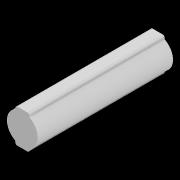
# Autodesk Inventor part: Axel_parametriserad_03
Saved by Autodesk Inventor 2020 (Build 240168000, 168)
## iProperties
Created: 2020-11-22
Part Number: Axel_parametriserad_03
Material: Generic
Document SubType Name: Modeling
Designer: Gottfrid
Density: 1 g/cm^3
Appearance: Default
Author: Gottfrid
Autodesk Inventor part; units mm, degrees
ref_plane "YZ Plane" through (0, 0, 0) normal (1, 0, 0) x (0, 1, 0)
ref_plane "XZ Plane" through (0, 0, 0) normal (0, 1, 0) x (-1, 0, 0)
ref_plane "XY Plane" through (0, 0, 0) normal (0, 0, 1) x (1, 0, 0)
sketch "Sketch1" plane through (0, 0, 0) normal (0, 0, 1) x (1, 0, 0)
  circle A0 centre (0, 0) radius 3.4
  line L0 (1.1333, -3.7357) -> (-1.1333, -3.7357)
  line L1 (-1.5333, -3.3357) -> (-1.5333, 3.3357)
  line L2 (-1.1333, 3.7357) -> (1.1333, 3.7357)
  line L3 (1.5333, 3.3357) -> (1.5333, -3.3357)
  line L4 (1.5333, -3.7357) -> (-1.5333, 3.7357) construction
  line L5 (-1.5333, -3.7357) -> (1.5333, 3.7357) construction
  arc A1 (-1.1333, 3.7357) -> (-1.5333, 3.3357) centre (-1.1333, 3.3357) ccw
  arc A2 (1.5333, 3.3357) -> (1.1333, 3.7357) centre (1.1333, 3.3357) ccw
  arc A3 (1.1333, -3.7357) -> (1.5333, -3.3357) centre (1.1333, -3.3357) ccw
  arc A4 (-1.5333, -3.3357) -> (-1.1333, -3.7357) centre (-1.1333, -3.3357) ccw
  point P0 (-1.5333, 3.0346)
  point P1 (-1.5333, -3.0346)
  point P2 (1.5333, -3.0346)
  point P3 (1.5333, 3.0346)
  point P4 (-0.9416, 2.2076)
  point P5 (-0.9416, -2.2076)
  point P6 (0.9416, -2.2076)
  point P7 (0.9416, 2.2076)
  dimension "d0" = 6.8
  dimension "d1" = 3.0667
  dimension "d2" = 7.4714
  dimension "d3" = 0.4
  constraints: 12 end point, 8 point on circle, 8 point on line, 8 tangent, 5 centre point, 3 equal radius, 2 midpoint, 2 parallel, 1 coincident, 1 horizontal, 1 perpendicular
  measures "d0" diameter of A0
  measures "d1" distance between parallel lines of L3 L1
  measures "d2" distance between parallel lines of L0 L2
  measures "d3" radius of A1
extrude "Extrusion1" add sketch "Sketch1" along normal blind 30
equation "\"d0\" = D_axel - d_toleransAxel"
equation "\"d3\" = r_filletAxel"
equation "\"d4\" = h_axel"
equation "\"D_axel\" = D_axel_1"
equation "\"d_axelRing\" = d_axelRing_1"
equation "\"r_filletAxel\" = r_filletAxel_1_2_3"
equation "\"d_toleransAxel\" = 0.2"
equation "\"h_axel\" = 30"
equation "\"D_axel_1\" = 7"
equation "\"d_axelRing_1\" = 3"
equation "\"r_filletAxel_1\" = r_filletAxel_1_2_3"
equation "\"r_filletAxel_1_2_3\" = 0.4"
body "Solid1"
